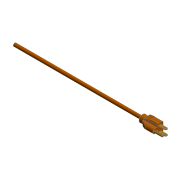
# Autodesk Inventor part: 576-070 PRODUCT D
Saved by Autodesk Inventor 2019.4 (Build 234330000, 330)
## iProperties
Created: 2005-11-09
Part Number: 576-070 PRODUCT D
Document SubType Name: Modeling
Designer: selting
Description: POWER CORD, 18/3 8FT, SJT
Material: Rubber (Orange Silicone)
Density: 0.93 g/cm^3
Appearance: Rubber (Orange)
Mass: 27.1689 g
Surface Area: 119.722 cm^2
Volume: 29.2138 cm^3
LOCATION: A8F
Source: B
MRP PLAN: P
UOM: EA
PRODUCT: GENERAL USE
QTYREQ: 1
Author: SELTING
Autodesk Inventor part; units mm, degrees
ref_plane "YZ Plane" through (0, 0, 0) normal (1, 0, 0) x (0, 1, 0)
ref_plane "XZ Plane" through (0, 0, 0) normal (0, 1, 0) x (-1, 0, 0)
ref_plane "XY Plane" through (0, 0, 0) normal (0, 0, 1) x (1, 0, 0)
sketch "Sketch1" plane through (0, 0, 0) normal (1, 0, 0) x (0, 1, 0)
  line L0 (-11.6205, 24.892) -> (11.6205, 24.892) construction
  line L1 (11.6205, 24.892) -> (11.6205, 0) construction
  line L2 (11.6205, 0) -> (-11.6205, 0) construction
  line L3 (-11.6205, 0) -> (-11.6205, 24.892) construction
  circle A0 centre (0, 19.4945) radius 5.3975 construction
  line L4 (-11.6205, 13.589) -> (11.6205, 13.589) construction
  line L5 (-5.3975, 19.4945) -> (-5.3975, 15.9702)
  line L6 (-7.7788, 13.589) -> (-9.2393, 13.589)
  line L7 (-11.6205, 11.2077) -> (-11.6205, 2.3812)
  line L8 (-9.2392, 0) -> (9.2392, 0)
  line L9 (11.6205, 2.3813) -> (11.6205, 11.2078)
  arc A1 (5.3975, 19.4945) -> (-5.3975, 19.4945) centre (0, 19.4945) ccw
  line L10 (-5.3975, 19.4945) -> (5.3975, 19.4945) construction
  line L11 (5.3975, 19.4945) -> (5.3975, 15.9702)
  line L12 (7.7788, 13.589) -> (9.2392, 13.589)
  arc A2 (-7.7788, 13.589) -> (-5.3975, 15.9702) centre (-7.7788, 15.9702) ccw
  arc A3 (5.3975, 15.9702) -> (7.7788, 13.589) centre (7.7788, 15.9703) ccw
  arc A4 (-9.2393, 13.589) -> (-11.6205, 11.2077) centre (-9.2393, 11.2077) ccw
  arc A5 (11.6205, 11.2078) -> (9.2392, 13.589) centre (9.2392, 11.2078) ccw
  arc A6 (-11.6205, 2.3812) -> (-9.2392, 0) centre (-9.2393, 2.3812) ccw
  arc A7 (9.2392, 0) -> (11.6205, 2.3813) centre (9.2392, 2.3813) ccw
  point P0 (0, 0)
  point P1 (0, 0)
  point P2 (0, 24.892)
  point P3 (-5.3975, 13.589)
  point P4 (5.3975, 13.589)
  dimension "d1" = 23.241
  dimension "d2" = 24.892
  dimension "d3" = 10.795
  dimension "d4" = 13.589
  dimension "d7" = 2.3813
  constraints: 26 end point, 17 point on circle, 16 point on line, 15 tangent, 8 centre point, 8 perpendicular, 6 equal radius, 2 coincident, 2 collinear, 2 midpoint, 2 parallel, 1 horizontal, 1 vertical alignment
  measures "d1" distance of L1.end L2.end
  measures "d2" distance of L0.end L1.end
  measures "d3" diameter of A0
  measures "d4" distance between parallel lines of L2 L4
  measures "d7" radius of A2
extrude "Extrusion1" add sketch "Sketch1" against normal blind 16.51
sketch "Sketch4" plane through (0, -9.2392, 0) normal (0, 0, -1) x (-1, 0, 0)
  line L0 (0, 0) -> (0, 18.4785) projected
  line L1 (16.51, -2.3813) -> (16.51, 0) construction
  line L2 (16.51, 18.4785) -> (16.51, 20.8597) construction
  line L3 (16.51, 20.8597) -> (31.115, 18.1292)
  line L4 (31.115, 18.1292) -> (31.115, 0.3492)
  line L5 (31.115, 0.3492) -> (16.51, -2.3813)
  line L6 (16.51, -2.3813) -> (16.51, 20.8597)
  point P0 (0, 9.2392)
  point P1 (0, 9.2392)
  point P2 (31.115, 9.2392)
  point P3 (0, 9.2392)
  dimension "d14" = 14.605
  dimension "d15" = 17.78
  constraints: 8 end point, 3 midpoint, 2 parallel, 1 horizontal alignment
  measures "d14" horizontal distance of L2.end L3.end
  measures "d15" distance of L3.end L4.end
extrude "Extrusion3" add sketch "Sketch4" against normal blind 25.4
sketch "Sketch5" plane through (0, -11.6205, 2.3812) normal (0, -1, 0) x (1, 0, 0)
  line L0 (-31.115, 23.0187) -> (-16.51, 23.0187) construction
  line L1 (-31.115, -2.3813) -> (-31.115, 23.0187) construction
  line L2 (-16.51, -2.3812) -> (-31.115, -2.3813) construction
  line L3 (-31.115, 15.3987) -> (-31.115, 23.0187)
  line L4 (-31.115, 23.0187) -> (-16.51, 23.0187)
  line L5 (-16.51, 23.0187) -> (-31.115, 15.3987)
  point P0 (0, -2.3813)
  dimension "d19" = 17.78
  constraints: 6 end point, 1 collinear, 1 perpendicular, 1 point on line
  measures "d19" distance of L1.start L3.start
extrude "Extrusion4" cut sketch "Sketch5" against normal through all
sketch "Sketch6" plane through (-16.51, -9.2393, 13.589) normal (1, 0, 0) x (0, 0, -1)
  arc A0 (0, 0) -> (2.3813, -2.3812) centre (2.3812, 0) ccw projected
  line L0 (0, 0) -> (0, 1.4605) projected
  arc A1 (0, 1.4605) -> (-2.3813, 3.8417) centre (-2.3813, 1.4605) ccw projected
  line L1 (-2.3813, 3.8417) -> (-5.9055, 3.8417) projected
  arc A2 (-5.9055, 14.6367) -> (-5.9055, 3.8417) centre (-5.9055, 9.2392) ccw projected
  arc A3 (2.3812, 20.8597) -> (0, 18.4785) centre (2.3812, 18.4785) ccw projected
  line L2 (0, 17.018) -> (0, 18.4785) projected
  arc A4 (-2.3813, 14.6368) -> (0, 17.018) centre (-2.3813, 17.018) ccw projected
  line L3 (-5.9055, 14.6367) -> (-2.3813, 14.6368) projected
  arc A5 (-5.9055, 14.6367) -> (-5.9055, 3.8417) centre (-5.9055, 9.2392) ccw projected
  line L4 (2.3812, 20.8597) -> (-11.811, 20.8597) projected
  line L5 (-11.811, -2.3813) -> (-11.811, 20.8597) projected
  line L6 (-11.811, -2.3813) -> (-11.811, 20.8597) projected
  line L7 (2.3813, -2.3812) -> (-11.811, -2.3813) projected
  arc A6 (11.2078, -2.3812) -> (13.589, 0) centre (11.2078, 0) ccw projected
  line L8 (13.589, -2.3812) -> (11.2078, -2.3812) projected
  line L9 (13.589, 0) -> (13.589, -2.3812) projected
  line L10 (13.589, 20.8598) -> (13.589, 18.4785) projected
  arc A7 (13.589, 18.4785) -> (11.2077, 20.8598) centre (11.2077, 18.4785) ccw projected
  line L11 (13.589, 20.8598) -> (11.2077, 20.8598) projected
  point P0 (13.589, 9.2393)
  point P1 (-11.43, 10.3188)
  constraints: 4 other
sketch "Sketch7" plane through (-31.115, -8.89, 0) normal (-1, 0, 0) x (0, 0, 1)
  line L0 (17.78, 0) -> (17.78, 17.78) construction
  line L1 (0, 17.78) -> (17.78, 17.78) construction
  line L2 (0, 0) -> (0, 17.78) construction
  line L3 (0, 0) -> (17.78, 0) construction
  circle A0 centre (7.9375, 8.89) radius 7.9375
  line L4 (0, 0) -> (0, 17.78) projected
  point P0 (0, 8.89)
  point P1 (0, 8.89)
  point P2 (0, 8.89)
  dimension "d24" = 15.875
  constraints: 2 horizontal alignment, 2 midpoint, 2 other
extrude "Extrusion6" add sketch "Sketch7" along normal blind 9.779 draft 4.5
sketch "Sketch9" plane through (-40.894, 0, 7.9375) normal (-1, 0, 0) x (0, 0, 1)
  circle A0 centre (0, 0) radius 3.81
  circle A1 centre (0, 0) radius 8.7071 construction
  dimension "d30" = 7.62
  constraints: 1 centre point, 1 coincident
  measures "d30" diameter of A0
extrude "Extrusion8" add sketch "Sketch9" along normal blind 304.8
sketch "Sketch10" plane through (0, 0, 0) normal (1, 0, 0) x (0, 0, -1)
  arc A0 (-18.161, 0) -> (-22.86, 0) centre (-20.5105, 0) ccw
  line L0 (-20.5105, 0) -> (-18.161, 0) construction
  line L1 (-20.5105, 0) -> (-22.86, 0) construction
  line L2 (-18.161, 0) -> (-22.86, 0)
  line L3 (-11.3792, 5.8293) -> (-5.08, 5.8293)
  line L4 (-5.08, 5.8293) -> (-5.08, 7.3025)
  line L5 (-5.08, 7.3025) -> (-11.3792, 7.3025)
  line L6 (-11.3792, 7.3025) -> (-11.3792, 5.8293)
  line L7 (0, -9.2392) -> (0, 9.2392) construction
  point P0 (0, 0)
  point P1 (-20.5105, 0)
  point P2 (0, 0)
  dimension "d37" = 2.3495
  dimension "d38" = 180
  dimension "d40" = 6.2992
  dimension "d42" = 1.4732
  dimension "d43" = 5.08
  dimension "d44" = 7.3025
  dimension "d45" = 17.78
  constraints: 14 end point, 2 horizontal, 2 midpoint, 2 parallel, 2 point on circle, 1 centre point, 1 horizontal alignment, 1 perpendicular
  measures "d37" radius of A0
  measures "d38" angle of L0 L1
  measures "d40" distance of L5.end L4.end
  measures "d42" distance between parallel lines of L3 L5
  measures "d43" distance between parallel lines of L7 L4
  measures "d44" distance from line of L5 point (0, 0)
  measures "d45" distance from line of L1.end L4
extrude "Extrusion9" add sketch "Sketch10" along normal blind 17.145 contours L6 L5 L4 L3
extrude "Extrusion10" add sketch "Sketch10" along normal blind 20.955 contours L2 A0
mirror "Mirror1" about plane through (0, 0, 0) normal (0, 1, 0) of "Extrusion10", "Extrusion9"
fillet "Fillet1" radius 2.3495 1 edges at (20.955, 0, 22.86)
sketch "Sketch11" plane through (0, 7.3025, 11.3792) normal (0, 1, 0) x (1, 0, 0)
  line L0 (0, 0) -> (0, 6.2992) construction
  line L1 (0, 0) -> (17.145, 0) construction
  line L2 (17.145, 6.2992) -> (17.145, 0) construction
  line L3 (0, 6.2992) -> (17.145, 6.2992) construction
  circle A0 centre (12.3825, 3.1496) radius 1.5875
  arc A1 (17.145, 1.5875) -> (15.5575, 0) centre (17.145, 0) ccw
  line L4 (17.145, 1.5875) -> (17.145, 0)
  line L5 (15.5575, 0) -> (17.145, 0)
  arc A2 (15.5575, 6.2992) -> (17.145, 4.7117) centre (17.145, 6.2992) ccw
  line L6 (17.145, 4.7117) -> (17.145, 6.2992)
  line L7 (17.145, 6.2992) -> (15.5575, 6.2992)
  point P0 (0, 11.3792)
  point P1 (17.145, 3.1496)
  dimension "d51" = 3.175
  dimension "d52" = 4.7625
  dimension "d53" = 1.5875
  constraints: 8 end point, 4 point on circle, 3 centre point, 3 perpendicular, 2 coincident, 2 point on line, 1 collinear, 1 equal radius, 1 horizontal alignment, 1 midpoint
  measures "d51" diameter of A0
  measures "d52" distance from line of L2 A0.centre
  measures "d53" distance from line of L5.start L4
extrude "Extrusion11" cut sketch "Sketch11" against normal through all
extrude "Extrusion12" cut sketch "Sketch6" against normal through all
sketch "Sketch12" plane through (-40.894, 0, 7.9375) normal (-1, 0, 0) x (0, 0, 1)
  circle A0 centre (0, 0) radius 7.9375 construction
  circle A1 centre (0, 0) radius 7.493
  point P0 (-7.9375, 0)
  dimension "d59" = 14.986
  constraints: 1 centre point, 1 coincident, 1 horizontal alignment
  measures "d59" diameter of A1
extrude "Extrusion13" add sketch "Sketch12" along normal blind 2.286
fillet "Fillet3" radius 2.032 1 edges at (-43.18, 0, 0.4445)
sketch "Sketch13" plane through (0, 0, 0) normal (1, 0, 0) x (0, 0, -1)
  line L0 (-15.3294, -3.9038) -> (-15.3294, -0.9424) construction
  line L1 (-15.3294, -0.9424) -> (-12.1544, -0.9424) construction
  line L2 (-12.1544, -0.9424) -> (-12.1544, -3.9038) construction
  line L3 (-12.1544, -3.9038) -> (-15.3294, -3.9038) construction
  spline S0 degree 2 poles (-13.7393, -1.0788) (-13.3045, -1.0788) (-12.6046, -1.4313) (-12.4091, -1.7271) knots 0 0 0 1 2 2 2
  spline S1 degree 2 poles (-12.4091, -1.7271) (-12.2573, -1.969) (-12.1544, -2.4656) (-12.1544, -2.8515) knots 0 0 0 1 2 2 2
  line L4 (-12.1544, -2.8515) -> (-12.1544, -3.5822)
  line L5 (-12.1544, -3.5822) -> (-15.3294, -3.5822)
  line L6 (-15.3294, -3.5822) -> (-15.3294, -2.8592)
  spline S2 degree 2 poles (-15.3294, -2.8592) (-15.3294, -2.4115) (-15.1956, -1.9021) (-15.0772, -1.722) knots 0 0 0 1 2 2 2
  spline S3 degree 2 poles (-15.0772, -1.722) (-14.874, -1.4158) (-14.2024, -1.0788) (-13.7393, -1.0788) knots 0 0 0 1 2 2 2
  spline S4 degree 2 poles (-13.7445, -1.5187) (-14.1098, -1.5187) (-14.627, -1.7606) (-14.7736, -1.9999) knots 0 0 0 1 2 2 2
  spline S5 degree 2 poles (-14.7736, -1.9999) (-14.874, -2.1697) (-14.964, -2.5531) (-14.964, -2.8386) knots 0 0 0 1 2 2 2
  line L7 (-14.964, -2.8386) -> (-14.964, -3.1603)
  line L8 (-14.964, -3.1603) -> (-12.5197, -3.1603)
  line L9 (-12.5197, -3.1603) -> (-12.5197, -2.8386)
  spline S6 degree 2 poles (-12.5197, -2.8386) (-12.5197, -2.5582) (-12.6098, -2.1337) (-12.7307, -1.9613) knots 0 0 0 1 2 2 2
  spline S7 degree 2 poles (-12.7307, -1.9613) (-12.8799, -1.74) (-13.374, -1.5187) (-13.7445, -1.5187) knots 0 0 0 1 2 2 2
  point P0 (0, 0)
  constraints: 2 other
emboss "Emboss1" sketch "Sketch13" operation cut depth 0.127 direction (-1, 0, 0)
body "Solid2"
